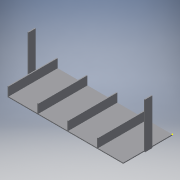
# Autodesk Inventor part: ModulePlate2.0
Saved by Autodesk Inventor 2016 (Build 200138000, 138)
## iProperties
Created: 2016-11-16
Part Number: ModulePlate2.0
Material: Generic
Document SubType Name: Modeling
Designer: RoboticsUser
Density: 1 g/cm^3
Appearance: Default
Mass: 39.7571 g
Surface Area: 509.371 cm^2
Volume: 39.7571 cm^3
Author: RoboticsUser
Autodesk Inventor part; units mm, degrees
ref_plane "YZ Plane" through (0, 0, 0) normal (1, 0, 0) x (0, 1, 0)
ref_plane "XZ Plane" through (0, 0, 0) normal (0, 1, 0) x (-1, 0, 0)
ref_plane "XY Plane" through (0, 0, 0) normal (0, 0, 1) x (1, 0, 0)
sketch "Sketch1" plane through (0, 0, 0) normal (0, 0, 1) x (1, 0, 0)
  line L0 (0, 0) -> (-203.2, 0)
  line L1 (-203.2, 0) -> (-203.2, -1.6002)
  line L2 (-203.2, -1.6002) -> (0, -1.6002)
  line L3 (0, -1.6002) -> (0, 0)
  dimension "d0" = 203.2
  dimension "d1" = 1.6002
  constraints: 8 end point, 2 parallel, 1 horizontal, 1 perpendicular
  measures "d0" distance of L2.end L1.end
  measures "d1" distance of L1.end L0.end
extrude "Extrusion1" add sketch "Sketch1" along normal blind 86.36
sketch "Sketch2" plane through (-203.2, 0, 0) normal (0, 1, 0) x (1, 0, 0)
  line L0 (203.2, 0) -> (0, 0) projected
  line L1 (203.2, -86.36) -> (0, -86.36) projected
  line L2 (0, 0) -> (1.6002, 0)
  line L3 (1.6002, 0) -> (1.6002, -86.36)
  line L4 (1.6002, -86.36) -> (0, -86.36)
  line L5 (0, -86.36) -> (0, 0)
  dimension "d4" = 1.6002
  constraints: 8 end point, 2 parallel, 1 horizontal, 1 perpendicular, 1 point on line
  measures "d4" distance of L3.end L4.end
extrude "Extrusion2" add sketch "Sketch2" along normal blind 15.24
sketch "Sketch3" plane through (0, 0, 86.36) normal (0, 1, 0) x (1, 0, 0)
  line L0 (-203.2, 0) -> (0, 0) projected
  line L1 (-203.2, 86.36) -> (0, 86.36) projected
  line L2 (-150.7998, 0) -> (-149.1996, 0)
  line L3 (-149.1996, 0) -> (-149.1996, 86.36)
  line L4 (-149.1996, 86.36) -> (-150.7998, 86.36)
  line L5 (-150.7998, 86.36) -> (-150.7998, 0)
  dimension "d7" = 1.6002
  constraints: 8 end point, 2 parallel, 2 point on line, 1 horizontal, 1 perpendicular
  measures "d7" distance of L4.end L3.end
extrude "Extrusion3" add sketch "Sketch3" along normal blind 15.24
sketch "Sketch4" plane through (0, 0, 86.36) normal (0, 1, 0) x (1, 0, 0)
  line L0 (-203.2, 0) -> (0, 0) projected
  line L1 (-203.2, 86.36) -> (0, 86.36) projected
  line L2 (-98.3996, 0) -> (-96.7994, 0)
  line L3 (-96.7994, 0) -> (-96.7994, 86.36)
  line L4 (-96.7994, 86.36) -> (-98.3996, 86.36)
  line L5 (-98.3996, 86.36) -> (-98.3996, 0)
  dimension "d10" = 1.6002
  constraints: 8 end point, 2 parallel, 2 point on line, 1 horizontal, 1 perpendicular
  measures "d10" distance of L4.end L3.end
extrude "Extrusion4" add sketch "Sketch4" along normal blind 15.24
sketch "Sketch5" plane through (0, 0, 86.36) normal (0, 1, 0) x (1, 0, 0)
  line L0 (0, 0) -> (-96.7994, 0) projected
  line L1 (0, 86.36) -> (-96.7994, 86.36) projected
  line L2 (-45.9994, 0) -> (-44.3992, 0)
  line L3 (-44.3992, 0) -> (-44.3992, 86.36)
  line L4 (-44.3992, 86.36) -> (-45.9994, 86.36)
  line L5 (-45.9994, 86.36) -> (-45.9994, 0)
  dimension "d13" = 1.6002
  constraints: 8 end point, 2 parallel, 2 point on line, 1 horizontal, 1 perpendicular
  measures "d13" distance of L4.end L3.end
extrude "Extrusion5" add sketch "Sketch5" along normal blind 15.24
sketch "Sketch6" plane through (-203.2, -1.6002, 0) normal (-1, 0, 0) x (0, 0, 1)
  line L0 (0, 0) -> (86.36, 0) projected
  line L1 (36.83, 0) -> (49.53, 0)
  line L2 (49.53, 0) -> (49.53, 80.01)
  line L3 (49.53, 80.01) -> (36.83, 80.01)
  line L4 (36.83, 80.01) -> (36.83, 0)
  point P0 (0, 1.6002)
  dimension "d16" = 12.7
  dimension "d17" = 80.01
  constraints: 8 end point, 2 parallel, 1 horizontal, 1 perpendicular, 1 point on line
  measures "d16" distance of L3.end L2.end
  measures "d17" distance of L2.end L1.end
extrude "Extrusion6" add sketch "Sketch6" along normal blind 1.6002
sketch "Sketch7" plane through (0, 0, 86.36) normal (1, 0, 0) x (0, 0, -1)
  line L0 (36.83, -1.6002) -> (0, -1.6002) projected
  line L1 (49.53, 78.4098) -> (49.53, -1.6002) projected
  line L2 (36.83, -1.6002) -> (49.53, -1.6002)
  line L3 (49.53, -1.6002) -> (49.53, 78.4098)
  line L4 (49.53, 78.4098) -> (36.83, 78.4098)
  line L5 (36.83, 78.4098) -> (36.83, -1.6002)
  point P0 (86.36, 0)
  dimension "d20" = 80.01
  constraints: 8 end point, 2 parallel, 1 horizontal, 1 perpendicular
  measures "d20" distance of L1.start L2.end
extrude "Extrusion7" add sketch "Sketch7" along normal blind 1.6002
sketch "Sketch8" plane through (-96.7994, 0, 86.36) normal (0, 1, 0) x (1, 0, 0)
  point P0 (96.7994, 86.36)
body "Solid1"
